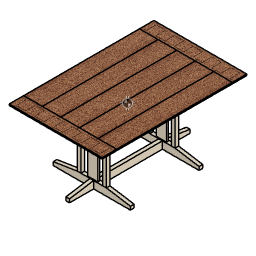
Trestle Table 2020 (Autodesk Fusion 360 design; units mm, degrees)
Autodesk Fusion 360 part; units mm, degrees
(part 1 of 2)
sketch "Sketch2" plane through (0, 0, 0) normal (1, 0, 0) x (0, 1, 0) in component "TopBoard"
  line L0 (0, 0) -> (1219.2, 0)
  line L1 (1219.2, 22.225) -> (0, 22.225)
  line L2 (609.6, 22.225) -> (609.6, 0) construction
  line L3 (0, 14.2875) -> (-25.4, 14.2875)
  line L4 (-25.4, 14.2875) -> (-25.4, 7.9375)
  line L5 (-25.4, 7.9375) -> (0, 7.9375)
  line L6 (0, 22.225) -> (0, 14.2875)
  line L7 (0, 7.9375) -> (0, 0)
  line L8 (1244.6, 14.2875) -> (1244.6, 7.9375)
  line L9 (1219.2, 22.225) -> (1219.2, 14.2875)
  line L10 (1244.6, 7.9375) -> (1219.2, 7.9375)
  line L11 (1219.2, 7.9375) -> (1219.2, 0)
  line L12 (1219.2, 14.2875) -> (1244.6, 14.2875)
  line L13 (1219.2, 0) -> (1219.2, 22.225) construction
  dimension "d18" = 1219.2
  dimension "d19" = 22.225
  dimension "d20" = 25.4
  dimension "d21" = 6.35
  constraint horizontal L0
  constraint horizontal L1
  constraint vertical L6
  constraint coincident L0.start L7.end
  constraint midpoint L1 L2.start
  constraint midpoint L0 L2.end
  constraint perpendicular L3 L6
  constraint perpendicular L3 L4
  constraint coincident L5.end L6
  constraint perpendicular L5 L6
  constraint collinear L6 L7
  constraint equal L6 L7
  constraint symmetric L0.start L2 L0.end
  constraint symmetric L1.end L2 L1.start
  constraint symmetric L2 L3.start L9.end
  constraint symmetric L2 L3.end L8.start
  constraint symmetric L2 L4.end L8.end
  constraint symmetric L2 L5.end L10.end
  constraint perpendicular L0 L13
  measures "d18" distance of L0.start L0.end
  measures "d19" distance of L0 L1
  measures "d20" distance of L3.start L3.end
  measures "d21" distance of L3.end L4.end
extrude "Extrude1" add sketch "Sketch2" along normal blind 195.58 makes body 1 in component "TopBoard"
ref_plane "WorkPlane1" through (97.79, 609.6, 11.1125) normal (0, -1, 0) x (0, 0, -1) in component "TopBoard"
sketch "Sketch3" plane through (0, -25.4, 0) normal (0, -1, 0) x (1, 0, 0) in component "TopBoard"
  line L0 (0, 14.2875) -> (0, 7.9375)
  line L1 (0, 7.9375) -> (195.58, 7.9375)
  line L2 (195.58, 7.9375) -> (195.58, 14.2875)
  line L3 (195.58, 14.2875) -> (0, 14.2875)
  line L4 (48.895, 14.2875) -> (146.685, 14.2875)
  line L5 (146.685, 14.2875) -> (146.685, 7.9375)
  line L6 (146.685, 7.9375) -> (48.895, 7.9375)
  line L7 (48.895, 7.9375) -> (48.895, 14.2875)
  dimension "d28" = 97.79
  constraint horizontal L4
  constraint vertical L5
  constraint horizontal L6
  constraint vertical L7
  constraint coincident L1 L5.end
  constraint coincident L3 L4.start
  constraint midpoint L3 L4
  measures "d28" distance of L4.start L4.end
extrude "Extrude2" add sketch "Sketch3" along normal blind 101.6 contours L1 L3 L4 L5 L6 L7 bodies 1 in component "TopBoard"
mirror "Mirror1" about plane through (97.79, 609.6, 11.1125) normal (0, -1, 0) of "Extrude2" in component "TopBoard"
sketch "Sketch4" plane through (0, 0, 0) normal (-1, 0, 0) x (0, -1, 0) in component "TopBoard"
  line L0 (0, 22.225) -> (-1219.2, 22.225)
  line L1 (-1219.2, 22.225) -> (-1219.2, 14.2875)
  line L2 (-1219.2, 14.2875) -> (-1244.6, 14.2875)
  line L3 (-1244.6, 14.2875) -> (-1244.6, 7.9375)
  line L4 (-1244.6, 7.9375) -> (-1219.2, 7.9375)
  line L5 (-1219.2, 7.9375) -> (-1219.2, 0)
  line L6 (-1219.2, 0) -> (0, 0)
  line L7 (0, 0) -> (0, 7.9375)
  line L8 (0, 7.9375) -> (25.4, 7.9375)
  line L9 (25.4, 7.9375) -> (25.4, 14.2875)
  line L10 (25.4, 14.2875) -> (0, 14.2875)
  line L11 (0, 14.2875) -> (0, 22.225)
  line L12 (-264.1209, 0) -> (-266.7, 7.9375)
  line L13 (-266.7, 7.9375) -> (-228.6, 7.9375)
  line L14 (-228.6, 7.9375) -> (-231.1791, 0)
  dimension "d61" = 38.1
  dimension "d62" = 108
  dimension "d63" = 108
  dimension "d64" = 7.9375
  dimension "d65" = 228.6
  constraint coincident L6 L12.start
  constraint parallel L6 L13
  constraint coincident L6 L14.end
  measures "d61" distance of L12.end L13.end
  measures "d62" angle of L6 L12
  measures "d63" angle of L6 L14
  measures "d64" distance of L6 L13
  measures "d65" distance of L7 L13.end
extrude "Extrude3" cut sketch "Sketch4" against normal up to surface (195.58 mm away) contours L6 L12 L13 L14 bodies 1 in component "TopBoard"
mirror "Mirror5" about plane through (97.79, 609.6, 11.1125) normal (0, -1, 0) of "Extrude3" in component "TopBoard"
pattern_linear "00000000-0000-0000-0000-000000000000" [suppressed]
sketch "Sketch2 (2)" plane through (0, 0, 0) normal (1, 0, 0) x (0, 1, 0) in component "TopBoard_Edge"
  line L0 (0, 0) -> (1219.2, 0)
  line L1 (1219.2, 22.225) -> (0, 22.225)
  line L2 (609.6, 22.225) -> (609.6, 0) construction
  line L3 (0, 14.2875) -> (-25.4, 14.2875)
  line L4 (-25.4, 14.2875) -> (-25.4, 7.9375)
  line L5 (-25.4, 7.9375) -> (0, 7.9375)
  line L6 (0, 22.225) -> (0, 14.2875)
  line L7 (0, 7.9375) -> (0, 0)
  line L8 (1244.6, 14.2875) -> (1244.6, 7.9375)
  line L9 (1219.2, 22.225) -> (1219.2, 14.2875)
  line L10 (1244.6, 7.9375) -> (1219.2, 7.9375)
  line L11 (1219.2, 7.9375) -> (1219.2, 0)
  line L12 (1219.2, 14.2875) -> (1244.6, 14.2875)
  line L13 (1219.2, 0) -> (1219.2, 22.225) construction
  dimension "d18_1" = 1219.2
  dimension "d19_1" = 22.225
  dimension "d20_1" = 25.4
  dimension "d21_1" = 6.35
  constraint horizontal L0
  constraint horizontal L1
  constraint vertical L6
  constraint coincident L0.start L7.end
  constraint midpoint L1 L2.start
  constraint midpoint L0 L2.end
  constraint perpendicular L3 L6
  constraint perpendicular L3 L4
  constraint coincident L5.end L6
  constraint perpendicular L5 L6
  constraint collinear L6 L7
  constraint equal L6 L7
  constraint symmetric L0.start L2 L0.end
  constraint symmetric L1.end L2 L1.start
  constraint symmetric L2 L3.start L9.end
  constraint symmetric L2 L3.end L8.start
  constraint symmetric L2 L4.end L8.end
  constraint symmetric L2 L5.end L10.end
  constraint perpendicular L0 L13
  measures "d18_1" distance of L0.start L0.end
  measures "d19_1" distance of L0 L1
  measures "d20_1" distance of L3.start L3.end
  measures "d21_1" distance of L3.end L4.end
extrude "Extrude1'" add sketch "Sketch2 (2)" along normal blind 195.58 separate body makes body 2 in component "TopBoard_Edge"
ref_plane "WorkPlane1" through (97.79, 609.6, 11.1125) normal (0, -1, 0) x (0, 0, -1) in component "TopBoard_Edge"
sketch "Sketch3 (2)" plane through (0, -25.4, 0) normal (0, -1, 0) x (1, 0, 0) in component "TopBoard_Edge"
  line L0 (0, 14.2875) -> (0, 7.9375)
  line L1 (0, 7.9375) -> (195.58, 7.9375)
  line L2 (195.58, 7.9375) -> (195.58, 14.2875)
  line L3 (195.58, 14.2875) -> (0, 14.2875)
  line L4 (48.895, 14.2875) -> (146.685, 14.2875)
  line L5 (146.685, 14.2875) -> (146.685, 7.9375)
  line L6 (146.685, 7.9375) -> (48.895, 7.9375)
  line L7 (48.895, 7.9375) -> (48.895, 14.2875)
  dimension "d28_1" = 97.79
  constraint horizontal L4
  constraint vertical L5
  constraint horizontal L6
  constraint vertical L7
  constraint coincident L1 L5.end
  constraint coincident L3 L4.start
  constraint midpoint L3 L4
  measures "d28_1" distance of L4.start L4.end
extrude "Extrude2'" add sketch "Sketch3 (2)" along normal blind 101.6 contours L1 L3 L4 L5 L6 L7 bodies 2 in component "TopBoard_Edge"
mirror "Mirror1'" about plane through (97.79, 609.6, 11.1125) normal (0, -1, 0) of "Extrude2'" in component "TopBoard_Edge"
sketch "Sketch4 (2)" plane through (0, 0, 0) normal (-1, 0, 0) x (0, -1, 0) in component "TopBoard_Edge"
  line L0 (0, 22.225) -> (-1219.2, 22.225)
  line L1 (-1219.2, 22.225) -> (-1219.2, 14.2875)
  line L2 (-1219.2, 14.2875) -> (-1244.6, 14.2875)
  line L3 (-1244.6, 14.2875) -> (-1244.6, 7.9375)
  line L4 (-1244.6, 7.9375) -> (-1219.2, 7.9375)
  line L5 (-1219.2, 7.9375) -> (-1219.2, 0)
  line L6 (-1219.2, 0) -> (0, 0)
  line L7 (0, 0) -> (0, 7.9375)
  line L8 (0, 7.9375) -> (25.4, 7.9375)
  line L9 (25.4, 7.9375) -> (25.4, 14.2875)
  line L10 (25.4, 14.2875) -> (0, 14.2875)
  line L11 (0, 14.2875) -> (0, 22.225)
  line L12 (-264.1209, 0) -> (-266.7, 7.9375)
  line L13 (-266.7, 7.9375) -> (-228.6, 7.9375)
  line L14 (-228.6, 7.9375) -> (-231.1791, 0)
  dimension "d61_1" = 38.1
  dimension "d62_1" = 108
  dimension "d63_1" = 108
  dimension "d64_1" = 7.9375
  dimension "d65_1" = 228.6
  constraint coincident L6 L12.start
  constraint parallel L6 L13
  constraint coincident L6 L14.end
  measures "d61_1" distance of L12.end L13.end
  measures "d62_1" angle of L6 L12
  measures "d63_1" angle of L6 L14
  measures "d64_1" distance of L6 L13
  measures "d65_1" distance of L7 L13.end
extrude "Extrude3'" cut sketch "Sketch4 (2)" against normal up to surface (195.58 mm away) contours L6 L12 L13 L14 bodies 2 in component "TopBoard_Edge"
mirror "Mirror5'" about plane through (97.79, 609.6, 11.1125) normal (0, -1, 0) of "Extrude3'" in component "TopBoard_Edge"
chamfer "Chamfer1" distance 50.1154 angle 9 3 edges at (0, 609.6, 0) (0, 115.5895, 0) (0, 1103.6105, 0) measured on face at (65.1933, 494.4403, 0) measured on face at (65.1933, 154.1194, 0) measured on face at (65.1933, 1065.0806, 0) on bodies 2 in component "TopBoard_Edge"
sketch "Sketch1" plane through (0, 0, 0) normal (1, 0, 0) x (0, 1, 0) in component "BreadBoard"
  line L0 (50.1154, 0) -> (152.4, 0)
  line L1 (152.4, 22.225) -> (0, 22.225)
  line L2 (0, 22.225) -> (0, 7.9375)
  line L3 (152.4, 14.2875) -> (127, 14.2875)
  line L4 (127, 14.2875) -> (127, 7.9375)
  line L5 (127, 7.9375) -> (152.4, 7.9375)
  line L6 (152.4, 0) -> (152.4, 7.9375)
  line L7 (152.4, 14.2875) -> (152.4, 22.225)
  line L8 (0, 7.9375) -> (50.1154, 0)
  dimension "d99" = 22.225
  dimension "d100" = 7.9375
  dimension "d103" = 152.4
  dimension "d104" = 6.35
  dimension "d105" = 25.4
  dimension "d596" = 99
  constraint horizontal L0
  constraint vertical L6
  constraint horizontal L1
  constraint vertical L2
  constraint coincident L3.start L6
  constraint perpendicular L3 L6
  constraint perpendicular L3 L4
  constraint perpendicular L5 L6
  constraint collinear L6 L7
  constraint equal L6 L7
  constraint coincident origin L2
  constraint coincident origin L0
  measures "d99" distance of origin L1.end
  measures "d100" distance of L0 L2.end
  measures "d103" distance of L1.start L1.end
  measures "d104" distance of L3.end L4.end
  measures "d105" distance of L3.start L3.end
  measures "d596" angle of L2 L8
extrude "Extrude1''" add sketch "Sketch1" along normal blind 977.9 separate body makes body 3 in component "BreadBoard"
sketch "Sketch2 (3)" plane through (0, 127, 0) normal (0, 1, 0) x (-1, 0, 0) in component "BreadBoard"
  line L0 (0, 7.9375) -> (0, 14.2875)
  line L1 (0, 14.2875) -> (-977.9, 14.2875)
  line L2 (-977.9, 14.2875) -> (-977.9, 7.9375)
  line L3 (-977.9, 7.9375) -> (0, 7.9375)
  line L4 (-146.685, 14.2875) -> (-48.895, 14.2875)
  line L5 (-48.895, 14.2875) -> (-48.895, 7.9375)
  line L6 (-48.895, 7.9375) -> (-146.685, 7.9375)
  line L7 (-146.685, 7.9375) -> (-146.685, 14.2875)
  line L8 (-342.265, 7.9375) -> (-342.265, 14.2875)
  line L9 (-244.475, 14.2875) -> (-244.475, 7.9375)
  line L10 (-244.475, 7.9375) -> (-342.265, 7.9375)
  line L11 (-342.265, 14.2875) -> (-244.475, 14.2875)
  line L12 (-537.845, 7.9375) -> (-537.845, 14.2875)
  line L13 (-440.055, 14.2875) -> (-440.055, 7.9375)
  line L14 (-440.055, 7.9375) -> (-537.845, 7.9375)
  line L15 (-537.845, 14.2875) -> (-440.055, 14.2875)
  line L16 (-733.425, 7.9375) -> (-733.425, 14.2875)
  line L17 (-635.635, 14.2875) -> (-635.635, 7.9375)
  line L18 (-635.635, 7.9375) -> (-733.425, 7.9375)
  line L19 (-733.425, 14.2875) -> (-635.635, 14.2875)
  line L20 (-929.005, 7.9375) -> (-929.005, 14.2875)
  line L21 (-831.215, 14.2875) -> (-831.215, 7.9375)
  line L22 (-831.215, 7.9375) -> (-929.005, 7.9375)
  line L23 (-929.005, 14.2875) -> (-831.215, 14.2875)
  dimension "d108" = 97.79
  dimension "d109" = 48.895
  dimension "d113" = 195.58
  dimension "d114" = 0
  constraint horizontal L4
  constraint vertical L5
  constraint horizontal L6
  constraint vertical L7
  constraint coincident L3 L5.end
  constraint coincident L1 L4.start
  measures "d108" distance of L4.start L4.end
  measures "d109" distance of L0 L5
extrude "Extrude2''" cut sketch "Sketch2 (3)" against normal blind 101.6 contours L1 L3 L4 L5 L6 L7 | L1 L3 L8 L9 L10 L11 | L1 L3 L12 L13 L14 L15 | L1 L3 L16 L17 L18 L19 | L1 L3 L20 L21 L22 L23 bodies 3 in component "BreadBoard"
sketch "Sketch3 (3)" plane through (0, 152.4, 0) normal (0, 1, 0) x (-1, 0, 0) in component "BreadBoard"
  line L0 (0, 0) -> (0, 7.9375)
  line L1 (0, 7.9375) -> (-977.9, 7.9375)
  line L2 (-977.9, 7.9375) -> (-977.9, 0)
  line L3 (-977.9, 0) -> (0, 0)
  line L4 (0, 7.9375) -> (-50.1154, 0)
  line L5 (0, 14.2875) -> (0, 7.9375)
  dimension "d118" = 7.9375
  dimension "d597" = 99
  constraint coincident L3 L4.end
  constraint coincident L0 L1.start
  measures "d118" distance of L0.start L0.end
  measures "d597" angle of L4 L5
ref_plane "WorkPlane1" through (488.95, 76.2, 11.1125) normal (-1, 0, 0) x (0, -1, 0) in component "BreadBoard"
extrude "Extrude3''" cut sketch "Sketch3 (3)" against normal up to surface (152.4 mm away) contours L0 L3 L4 bodies 3 in component "BreadBoard"
mirror "Mirror1''" about plane through (488.95, 76.2, 11.1125) normal (-1, 0, 0) of "Extrude3''" in component "BreadBoard"
sketch "Sketch1 (2)" plane through (0, 0, 0) normal (1, 0, 0) x (0, 1, 0) in component "TrestleTop"
  line L0 (0, 0) -> (38.1, 0)
  line L1 (38.1, 0) -> (38.1, 76.2)
  line L2 (0, 76.2) -> (0, 0)
  line L3 (38.1, 76.2) -> (35.5209, 76.2)
  line L4 (2.5791, 76.2) -> (0, 76.2)
  line L5 (2.5791, 76.2) -> (0, 84.1375)
  line L6 (0, 84.1375) -> (38.1, 84.1375)
  line L7 (38.1, 84.1375) -> (35.5209, 76.2)
  dimension "d146" = 76.2
  dimension "d147" = 38.1
  dimension "d148" = 7.9375
  dimension "d149" = 72
  constraint horizontal L0
  constraint vertical L1
  constraint horizontal L3
  constraint vertical L2
  constraint coincident L0.start L2.end
  constraint coincident L4.start L3
  constraint collinear L3 L4
  constraint equal L3 L4
  constraint parallel L4 L6
  constraint coincident L1 L6.end
  constraint coincident L2 L5.end
  measures "d146" distance of L0.start L2.start
  measures "d147" distance of L0.start L0.end
  measures "d148" distance of L4 L6
  measures "d149" angle of L5 L6
extrude "Extrude1'''" add sketch "Sketch1 (2)" along normal blind 812.8 separate body makes body 4 in component "TrestleTop"
sketch "Sketch2 (4)" plane through (0, 0, 0) normal (0, -1, 0) x (1, 0, 0) in component "TrestleTop"
  line L0 (0, 76.2) -> (0, 0)
  line L1 (0, 0) -> (812.8, 0)
  line L2 (812.8, 0) -> (812.8, 76.2)
  line L3 (812.8, 76.2) -> (0, 76.2)
  line L4 (0, 40.2296) -> (254, 0)
  line L5 (406.4, 76.2) -> (406.4, 0) construction
  line L6 (812.8, 40.2296) -> (558.8, 0)
  dimension "d158" = 9
  dimension "d159" = 304.8
  dimension "d161" = 35.9704
  constraint coincident L0 L4.start
  constraint coincident L1 L4.end
  constraint midpoint L3 L5.start
  constraint midpoint L1 L5.end
  constraint symmetric L4.start L5 L6.start
  constraint symmetric L4.end L5 L6.end
  measures "d158" angle of L1 L4
  measures "d159" distance of L4.end L6.end
  measures "d161" distance of L0.start L4.start
extrude "Extrude2'''" cut sketch "Sketch2 (4)" against normal up to surface (38.1 mm away) contours L0 L1 L4 | L1 L2 L6 bodies 4 in component "TrestleTop"
sketch "Sketch3 (4)" plane through (0, 0, 0) normal (0, 0, -1) x (1, 0, 0) in component "TrestleTop"
  line L0 (254, 0) -> (254, -38.1)
  line L1 (254, -38.1) -> (558.8, -38.1)
  line L2 (558.8, -38.1) -> (558.8, 0)
  line L3 (558.8, 0) -> (254, 0)
  line L4 (260.35, -12.7) -> (285.75, -12.7)
  line L5 (285.75, -12.7) -> (285.75, -25.4)
  line L6 (285.75, -25.4) -> (260.35, -25.4)
  line L7 (260.35, -25.4) -> (260.35, -12.7)
  line L8 (285.7253, 0) -> (285.7747, -38.1) construction
  line L9 (406.4, 0) -> (406.4, -38.1) construction
  line L10 (552.45, -12.7) -> (527.05, -12.7)
  line L11 (552.45, -25.4) -> (552.45, -12.7)
  line L12 (527.05, -25.4) -> (552.45, -25.4)
  line L13 (527.05, -12.7) -> (527.05, -25.4)
  line L14 (355.9175, -12.7) -> (456.8825, -12.7)
  line L15 (456.8825, -12.7) -> (456.8825, -25.4)
  line L16 (456.8825, -25.4) -> (355.9175, -25.4)
  line L17 (355.9175, -25.4) -> (355.9175, -12.7)
  line L18 (456.8825, -12.7) -> (355.9175, -25.4) construction
  dimension "d162" = 6.35
  dimension "d163" = 25.4
  dimension "d164" = 12.7
  dimension "d592" = 12.7
  dimension "d593" = 100.965
  constraint vertical L5
  constraint vertical L7
  constraint coincident L3 L8.start
  constraint coincident L1 L8.end
  constraint midpoint L5 L8
  constraint midpoint L3 L9.start
  constraint midpoint L1 L9.end
  constraint symmetric L4.start L9 L10.start
  constraint symmetric L4.end L9 L10.end
  constraint symmetric L5.end L9 L12.start
  constraint symmetric L6.end L9 L11.start
  constraint horizontal L14
  constraint vertical L15
  constraint horizontal L16
  constraint vertical L17
  constraint midpoint L9 L18
  constraint horizontal L4
  constraint horizontal L6
  measures "d162" distance of L0 L7
  measures "d163" distance of L4.start L4.end
  measures "d164" distance of L4.start L6.end
  measures "d592" distance of L14.end L15.end
  measures "d593" distance of L14.start L14.end
extrude "Extrude3'''" cut sketch "Sketch3 (4)" against normal blind 38.1 contours L4 L5 L6 L7 | L10 L11 L12 L13 bodies 4 in component "TrestleTop"
sketch "Sketch1 (3)" plane through (0, 0, 0) normal (0, 0, 1) x (1, 0, 0) in component "TrestlePost"
  line L0 (0, 0) -> (38.1, 0)
  line L1 (38.1, 0) -> (38.1, 38.1)
  line L2 (38.1, 38.1) -> (0, 38.1)
  line L3 (0, 38.1) -> (0, 0)
  dimension "d199" = 38.1
  constraint horizontal L0
  constraint vertical L1
  constraint horizontal L2
  constraint vertical L3
  constraint coincident L0.start L3.end
  constraint equal L1 L2
  measures "d199" distance of L0.end L1.end
extrude "Extrude1''''" add sketch "Sketch1 (3)" along normal blind 536.575 separate body makes body 5 in component "TrestlePost"
ref_plane "WorkPlane1" through (19.05, 19.05, 268.2875) normal (0, 0, 1) x (1, 0, 0) in component "TrestlePost"
sketch "Sketch2 (5)" plane through (0, 0, 536.575) normal (0, 0, 1) x (-1, 0, 0) in component "TrestlePost"
  line L0 (0, -38.1) -> (0, 0)
  line L1 (0, 0) -> (-38.1, 0)
  line L2 (-38.1, 0) -> (-38.1, -38.1)
  line L3 (-38.1, -38.1) -> (0, -38.1)
  line L4 (-6.35, -25.4) -> (-31.75, -25.4)
  line L5 (-31.75, -25.4) -> (-31.75, -12.7)
  line L6 (-31.75, -12.7) -> (-6.35, -12.7)
  line L7 (-6.35, -12.7) -> (-6.35, -25.4)
  line L8 (0, -38.1) -> (-38.1, 0) construction
  line L9 (-31.75, -25.4) -> (-6.35, -12.7) construction
  dimension "d202" = 12.7
  dimension "d203" = 6.35
  constraint horizontal L4
  constraint vertical L5
  constraint horizontal L6
  constraint vertical L7
  constraint coincident L0.start L3.end
  constraint coincident L1.end L2.start
  constraint midpoint L8 L9
  measures "d202" distance of L4.end L5.end
  measures "d203" distance of L2 L5
extrude "Extrude2''''" add sketch "Sketch2 (5)" along normal blind 38.1 contours L4 L5 L6 L7 bodies 5 in component "TrestlePost"
mirror "Mirror1'''" about plane through (19.05, 19.05, 268.2875) normal (0, 0, 1) of "Extrude2''''" in component "TrestlePost"
sketch "Sketch1 (4)" plane through (0, 0, 0) normal (1, 0, 0) x (0, 1, 0) in component "TrestleBase"
  line L0 (0, 0) -> (38.1, 0)
  line L1 (38.1, 0) -> (38.1, 76.2)
  line L2 (0, 76.2) -> (0, 0)
  line L3 (38.1, 76.2) -> (0, 76.2)
  dimension "d146_1" = 76.2
  dimension "d147_1" = 38.1
  dimension "d572" = 0
  dimension "d573" = 0
  dimension "d574" = 0
  dimension "d575" = 0
  dimension "d584" = 0
  dimension "d585" = 0
  dimension "d586" = 0
  dimension "d587" = 0
  constraint horizontal L0
  constraint vertical L1
  constraint vertical L2
  constraint coincident L0.start L2.end
  constraint horizontal L3
  measures "d146_1" distance of L0.start L2.start
  measures "d147_1" distance of L0.start L0.end
extrude "Extrude1'''''" add sketch "Sketch1 (4)" along normal blind 812.8 separate body makes body 6 in component "TrestleBase"
sketch "Sketch2 (6)" plane through (0, 0, 0) normal (0, -1, 0) x (1, 0, 0) in component "TrestleBase"
  line L0 (0, 76.2) -> (0, 0)
  line L1 (0, 0) -> (812.8, 0)
  line L2 (812.8, 0) -> (812.8, 76.2)
  line L3 (0, 40.2296) -> (254, 0)
  line L4 (406.4, 76.2) -> (406.4, 0) construction
  line L5 (812.8, 40.2296) -> (558.8, 0)
  line L6 (812.8, 76.2) -> (0, 76.2)
  line L7 (425.45, 76.2) -> (425.45, 38.1)
  line L8 (425.45, 38.1) -> (387.35, 38.1)
  line L9 (387.35, 38.1) -> (387.35, 76.2)
  dimension "d158_1" = 9
  dimension "d159_1" = 304.8
  dimension "d161_1" = 35.9704
  dimension "d628" = 38.1
  constraint coincident L0 L3.start
  constraint coincident L1 L3.end
  constraint midpoint L1 L4.end
  constraint symmetric L3.start L4 L5.start
  constraint symmetric L3.end L4 L5.end
  constraint coincident L1 L5.end
  constraint coincident L6 L7.start
  constraint perpendicular L6 L7
  constraint perpendicular L7 L8
  constraint coincident L6 L9.end
  constraint perpendicular L6 L9
  constraint midpoint L4 L8
  constraint coincident L4.start L6
  measures "d158_1" angle of L1 L3
  measures "d159_1" distance of L3.end L5.end
  measures "d161_1" distance of L0.start L3.start
  measures "d628" distance of L7.start L9.end
extrude "Extrude2'''''" cut sketch "Sketch2 (6)" against normal up to surface (38.1 mm away) contours L0 L1 L3 | L6 L7 L8 L9 | L1 L2 L5 bodies 6 in component "TrestleBase"
sketch "Sketch3 (5)" plane through (0, 0, 0) normal (0, 0, -1) x (1, 0, 0) in component "TrestleBase"
  line L0 (254, 0) -> (254, -38.1)
  line L1 (254, -38.1) -> (558.8, -38.1)
  line L2 (558.8, -38.1) -> (558.8, 0)
  line L3 (558.8, 0) -> (254, 0)
  line L4 (260.35, -12.7) -> (285.75, -12.7)
  line L5 (285.75, -12.7) -> (285.75, -25.4)
  line L6 (285.75, -25.4) -> (260.35, -25.4)
  line L7 (260.35, -25.4) -> (260.35, -12.7)
  line L8 (285.7946, 0) -> (285.7054, -38.1) construction
  line L9 (406.4, 0) -> (406.4, -38.1) construction
  line L10 (552.45, -12.7) -> (527.05, -12.7)
  line L11 (552.45, -25.4) -> (552.45, -12.7)
  line L12 (527.05, -25.4) -> (552.45, -25.4)
  line L13 (527.05, -12.7) -> (527.05, -25.4)
  line L14 (355.9175, -12.7) -> (456.8825, -12.7)
  line L15 (456.8825, -12.7) -> (456.8825, -25.4)
  line L16 (456.8825, -25.4) -> (355.9175, -25.4)
  line L17 (355.9175, -25.4) -> (355.9175, -12.7)
  line L18 (456.8825, -12.7) -> (355.9175, -25.4) construction
  dimension "d162_1" = 6.35
  dimension "d163_1" = 25.4
  dimension "d164_1" = 12.7
  dimension "d559" = 100.965
  dimension "d560" = 12.7
  constraint vertical L5
  constraint vertical L7
  constraint coincident L3 L8.start
  constraint coincident L1 L8.end
  constraint midpoint L5 L8
  constraint midpoint L3 L9.start
  constraint midpoint L1 L9.end
  constraint symmetric L4.start L9 L10.start
  constraint symmetric L4.end L9 L10.end
  constraint symmetric L5.end L9 L12.start
  constraint symmetric L6.end L9 L11.start
  constraint horizontal L14
  constraint vertical L15
  constraint horizontal L16
  constraint vertical L17
  constraint horizontal L4
  constraint horizontal L6
  constraint midpoint L9 L18
  measures "d162_1" distance of L0 L7
  measures "d163_1" distance of L4.start L4.end
  measures "d164_1" distance of L4.start L6.end
  measures "d559" distance of L14.start L14.end
  measures "d560" distance of L14.end L15.end
extrude "Extrude3''''" cut sketch "Sketch3 (5)" against normal blind 38.1 contours L4 L5 L6 L7 | L10 L11 L12 L13 bodies 6 in component "TrestleBase"
sketch "Sketch3 (6)" plane through (0, 0, 0) normal (0, -1, 0) x (1, 0, 0) in component "TrestlePost"
  line L0 (0, 0) -> (38.1, 0)
  line L1 (38.1, 0) -> (38.1, 536.575)
  line L2 (38.1, 536.575) -> (0, 536.575)
  line L3 (0, 536.575) -> (0, 0)
  line L4 (12.7, 479.425) -> (25.4, 479.425)
  line L5 (25.4, 479.425) -> (25.4, 377.825)
  line L6 (25.4, 377.825) -> (12.7, 377.825)
  line L7 (12.7, 377.825) -> (12.7, 479.425)
  line L8 (0, 479.425) -> (38.1, 479.425) construction
  dimension "d337" = 12.7
  dimension "d338" = 101.6
  dimension "d339" = 377.825
  constraint horizontal L4
  constraint vertical L5
  constraint horizontal L6
  constraint vertical L7
  constraint coincident L3 L8.start
  constraint coincident L1 L8.end
  constraint perpendicular L1 L8
  constraint midpoint L4 L8
  measures "d337" distance of L4.start L4.end
  measures "d338" distance of L4.start L6.end
  measures "d339" distance of L0 L6
extrude "Extrude3'''''" cut sketch "Sketch3 (6)" against normal up to surface (38.1 mm away) contours L4 L5 L6 L7 bodies 5 in component "TrestlePost"
sketch "Sketch1 (5)" plane through (0, 0, 0) normal (0, 1, 0) x (1, 0, 0) in component "Stretcher"
  line L0 (0, 0) -> (19.304, 0)
  line L1 (19.304, 0) -> (19.304, -114.3)
  line L2 (19.304, -114.3) -> (0, -114.3)
  line L3 (0, -114.3) -> (0, 0)
  dimension "d366" = 19.304
  dimension "d367" = 114.3
  constraint horizontal L0
  constraint vertical L1
  constraint horizontal L2
  constraint vertical L3
  constraint coincident L0.start L3.end
  measures "d366" distance of L0.start L0.end
  measures "d367" distance of L0.start L2.end
extrude "Extrude1''''''" add sketch "Sketch1 (5)" along normal blind 685.8 separate body makes body 7 in component "Stretcher"
ref_plane "WorkPlane1" through (9.652, 342.9, 57.15) normal (0, 1, 0) x (0, 0, 1) in component "Stretcher"
sketch "Sketch2 (7)" plane through (0, 0, 0) normal (0, -1, 0) x (1, 0, 0) in component "Stretcher"
  line L0 (19.304, 114.3) -> (0, 114.3)
  line L1 (0, 114.3) -> (0, 0)
  line L2 (0, 0) -> (19.304, 0)
  line L3 (19.304, 0) -> (19.304, 114.3)
  line L4 (3.302, 107.95) -> (16.002, 107.95)
  line L5 (16.002, 107.95) -> (16.002, 6.35)
  line L6 (16.002, 6.35) -> (3.302, 6.35)
  line L7 (3.302, 6.35) -> (3.302, 107.95)
  line L8 (0, 114.3) -> (19.304, 0) construction
  line L9 (3.302, 6.35) -> (16.002, 107.95) construction
  dimension "d370" = 6.35
  dimension "d372" = 12.7
  constraint horizontal L4
  constraint vertical L5
  constraint horizontal L6
  constraint vertical L7
  constraint coincident L0.end L1.start
  constraint coincident L2.end L3.start
  constraint midpoint L8 L9
  measures "d370" distance of L0 L4
  measures "d372" distance of L4.start L4.end
extrude "Extrude2''''''" add sketch "Sketch2 (7)" along normal blind 38.1 contours L4 L5 L6 L7 bodies 7 in component "Stretcher"
ref_plane "WorkPlane2" through (9.652, -19.05, 57.15) normal (1, 0, 0) x (0, 0, 1) in component "Stretcher"
sketch "Sketch3 (7)" plane through (9.652, -50.8, 38.1) normal (1, 0, 0) x (0, 1, 0) in component "Stretcher"
  line L0 (50.8, 69.85) -> (12.7, 69.85)
  line L1 (50.8, -31.75) -> (12.7, -31.75)
  line L2 (12.7, 69.85) -> (12.7, -31.75)
  line L3 (12.7, -31.75) -> (0, -31.75)
  line L4 (0, -31.75) -> (-7.9961, 69.85)
  line L5 (-7.9961, 69.85) -> (12.7, 69.85)
  line L6 (50.8, 76.2) -> (50.8, -38.1)
  dimension "d400" = 38.1
  dimension "d401" = 4.5
  dimension "d404" = 12.7
  constraint coincident L0 L2.start
  constraint coincident L1 L2.end
  constraint perpendicular L1 L2
  constraint coincident L0 L4.end
  constraint coincident L1 L3.end
  measures "d400" distance of L2 L6
  measures "d401" angle of L2 L4
  measures "d404" distance of L1.end L3.end
mirror "Mirror2" about plane through (9.652, 342.9, 57.15) normal (0, 1, 0) of "Extrude2''''''" in component "Stretcher"
sketch "Sketch1 (6)" plane through (0, 0, 0) normal (0, 1, 0) x (1, 0, 0) in component "Panel"
  line L0 (140.97, 76.2) -> (445.77, 76.2)
  line L1 (140.97, 612.775) -> (445.77, 612.775)
  line L2 (252.9511, 76.2) -> (360.2661, 76.2)
  line L3 (360.2661, 76.2) -> (360.2661, 612.775)
  line L4 (360.2661, 612.775) -> (252.9511, 612.775)
  line L5 (252.9511, 612.775) -> (252.9511, 76.2)
  dimension "d530" = 107.315
  dimension "d568" = 0
  dimension "d569" = 0
  dimension "d570" = 0
  dimension "d571" = 0
  dimension "d580" = 0
  dimension "d581" = 0
  dimension "d582" = 0
  dimension "d583" = 0
  constraint horizontal L2
  constraint vertical L3
  constraint horizontal L4
  constraint vertical L5
  constraint coincident L1 L3.end
  constraint coincident L0 L2.start
  measures "d530" distance of L3.end L4.end
extrude "Extrude1'''''''" add sketch "Sketch1 (6)" along normal blind 19.304 separate body makes body 8 in component "Panel"
ref_plane "WorkPlane1" through (306.6086, 9.652, -344.4875) normal (0, 0, 1) x (1, 0, 0) in component "Panel"
sketch "Sketch2 (8)" plane through (0, 0, -76.2) normal (0, 0, 1) x (-1, 0, 0) in component "Panel"
  line L0 (-252.9511, 0) -> (-360.2661, 0)
  line L1 (-360.2661, 0) -> (-360.2661, -19.304)
  line L2 (-360.2661, -19.304) -> (-252.9511, -19.304)
  line L3 (-252.9511, -19.304) -> (-252.9511, 0)
  line L4 (-256.1261, -16.002) -> (-357.0911, -16.002)
  line L5 (-357.0911, -16.002) -> (-357.0911, -3.302)
  line L6 (-357.0911, -3.302) -> (-256.1261, -3.302)
  line L7 (-256.1261, -3.302) -> (-256.1261, -16.002)
  line L8 (-256.1261, -3.302) -> (-357.0911, -16.002) construction
  line L9 (-306.6086, -19.304) -> (-306.6086, 0) construction
  dimension "d561" = 12.7
  dimension "d562" = 3.175
  constraint horizontal L4
  constraint vertical L5
  constraint horizontal L6
  constraint vertical L7
  constraint midpoint L2 L9.start
  constraint midpoint L0 L9.end
  constraint midpoint L8 L9
  measures "d561" distance of L4.end L5.end
  measures "d562" distance of L3 L7
extrude "Extrude2'''''''" add sketch "Sketch2 (8)" along normal blind 6.35 contours L4 L5 L6 L7 bodies 8 in component "Panel"
mirror "Mirror1''''" about plane through (306.6086, 9.652, -344.4875) normal (0, 0, 1) of "Extrude2'''''''" in component "Panel"
sketch "Sketch2 (9)" plane through (0, 0, 0) normal (0, 1, 0) x (1, 0, 0)
  line L0 (-113.03, 688.975) -> (293.37, 73.1846)
  line L1 (312.42, 688.975) -> (699.77, 688.975)
  line L2 (-113.03, 688.975) -> (274.32, 688.975)
extrude "Extrude4" cut sketch "Sketch3 (4)" against normal blind 6.35 contours L14 L15 L16 L17 bodies 4 in component "TrestleTop"
extrude "Extrude4'" cut sketch "Sketch3 (5)" against normal blind 6.35 contours L14 L15 L16 L17 bodies 6 in component "TrestleBase"
sketch "Sketch1 (7)" plane through (0, 0, 0) normal (1, 0, 0) x (0, 1, 0) in component "FloorStretcher"
  line L0 (0, 0) -> (1270, 0)
  line L1 (1270, 0) -> (1270, 35.9704)
  line L2 (1270, 35.9704) -> (1016, 76.2)
  line L3 (1016, 76.2) -> (1016, 38.1)
  line L4 (1016, 38.1) -> (977.9, 38.1)
  line L5 (977.9, 38.1) -> (977.9, 76.2)
  line L6 (977.9, 76.2) -> (292.1, 76.2)
  line L7 (292.1, 76.2) -> (292.1, 38.1)
  line L8 (292.1, 38.1) -> (254, 38.1)
  line L9 (254, 38.1) -> (254, 76.2)
  line L10 (254, 76.2) -> (0, 35.9704)
  line L11 (0, 35.9704) -> (0, 0)
  line L12 (1270, 35.9704) -> (0, 35.9704) construction
  line L13 (635, 76.2) -> (635, 0) construction
  dimension "d620" = 38.1
  dimension "d621" = 1270
  dimension "d622" = 38.1
  dimension "d623" = 9
  dimension "d624" = 76.2
  dimension "d625" = 762
  constraint coincident L0.start L11.end
  constraint horizontal L0
  constraint perpendicular L0 L1
  constraint perpendicular L3 L4
  constraint perpendicular L4 L5
  constraint perpendicular L3 L6
  constraint perpendicular L6 L7
  constraint perpendicular L7 L8
  constraint perpendicular L8 L9
  constraint horizontal L12
  constraint vertical L11
  constraint collinear L4 L8
  constraint equal L4 L8
  constraint midpoint L6 L13.start
  constraint midpoint L0 L13.end
  constraint vertical L13
  constraint coincident L2.end L6
  constraint coincident L6 L9.end
  measures "d620" distance of L0 L8
  measures "d621" distance of L0.start L0.end
  measures "d622" distance of L3.end L4.end
  measures "d623" angle of L10 L12
  measures "d624" distance of L0 L6
  measures "d625" distance of L2.end L9.end
extrude "Extrude1''''''''" add sketch "Sketch1 (7)" along normal blind 38.1 separate body makes body 9 in component "FloorStretcher"
sketch "Sketch3 (8)" plane through (0, 19.304, 0) normal (0, 1, 0) x (-1, 0, 0) in component "Panel"
  line L0 (-252.9511, -612.775) -> (-252.9511, -76.2)
  line L1 (-252.9511, -76.2) -> (-360.2661, -76.2)
  line L2 (-360.2661, -76.2) -> (-360.2661, -612.775)
  line L3 (-360.2661, -612.775) -> (-252.9511, -612.775)
  line L4 (-306.6086, -88.9) -> (-347.5661, -129.8575)
  line L5 (-347.5661, -129.8575) -> (-306.6086, -170.815)
  line L6 (-306.6086, -170.815) -> (-265.6511, -129.8575)
  line L7 (-265.6511, -129.8575) -> (-306.6086, -88.9)
  line L8 (-281.2086, -88.9) -> (-265.6511, -88.9)
  line L9 (-265.6511, -88.9) -> (-265.6511, -104.4575)
  line L10 (-265.6511, -104.4575) -> (-281.2086, -88.9)
  line L11 (-306.6086, -76.2) -> (-306.6086, -612.775) construction
  line L12 (-265.6511, -155.2575) -> (-293.9086, -183.515)
  line L13 (-293.9086, -183.515) -> (-265.6511, -211.7725)
  line L14 (-265.6511, -211.7725) -> (-265.6511, -155.2575)
  line L15 (-360.2661, -344.4875) -> (-252.9511, -344.4875) construction
  line L16 (-306.6086, -278.13) -> (-265.6511, -237.1725)
  line L17 (-347.5661, -237.1725) -> (-306.6086, -278.13)
  line L18 (-306.6086, -196.215) -> (-347.5661, -237.1725)
  line L19 (-265.6511, -237.1725) -> (-306.6086, -196.215)
  line L20 (-306.6086, -385.445) -> (-265.6511, -344.4875)
  line L21 (-347.5661, -344.4875) -> (-306.6086, -385.445)
  line L22 (-306.6086, -303.53) -> (-347.5661, -344.4875)
  line L23 (-265.6511, -344.4875) -> (-306.6086, -303.53)
  line L24 (-306.6086, -492.76) -> (-265.6511, -451.8025)
  line L25 (-347.5661, -451.8025) -> (-306.6086, -492.76)
  line L26 (-306.6086, -410.845) -> (-347.5661, -451.8025)
  line L27 (-265.6511, -451.8025) -> (-306.6086, -410.845)
  line L28 (-265.6511, -319.0875) -> (-265.6511, -262.5725)
  line L29 (-265.6511, -262.5725) -> (-293.9086, -290.83)
  line L30 (-293.9086, -290.83) -> (-265.6511, -319.0875)
  line L31 (-265.6511, -426.4025) -> (-265.6511, -369.8875)
  line L32 (-265.6511, -369.8875) -> (-293.9086, -398.145)
  line L33 (-293.9086, -398.145) -> (-265.6511, -426.4025)
  line L34 (-265.6511, -533.7175) -> (-265.6511, -477.2025)
  line L35 (-265.6511, -477.2025) -> (-293.9086, -505.46)
  line L36 (-293.9086, -505.46) -> (-265.6511, -533.7175)
  line L37 (-306.6086, -600.075) -> (-265.6511, -559.1175)
  line L38 (-347.5661, -559.1175) -> (-306.6086, -600.075)
  line L39 (-306.6086, -518.16) -> (-347.5661, -559.1175)
  line L40 (-265.6511, -559.1175) -> (-306.6086, -518.16)
  line L41 (-281.2086, -600.075) -> (-265.6511, -600.075)
  line L42 (-265.6511, -584.5175) -> (-281.2086, -600.075)
  line L43 (-265.6511, -600.075) -> (-265.6511, -584.5175)
  line L44 (-347.5661, -477.2025) -> (-319.3086, -505.46)
  line L45 (-347.5661, -426.4025) -> (-347.5661, -369.8875)
  line L46 (-347.5661, -369.8875) -> (-319.3086, -398.145)
  line L47 (-332.0086, -600.075) -> (-347.5661, -600.075)
  line L48 (-347.5661, -533.7175) -> (-347.5661, -477.2025)
  line L49 (-319.3086, -505.46) -> (-347.5661, -533.7175)
  line L50 (-347.5661, -211.7725) -> (-347.5661, -155.2575)
  line L51 (-347.5661, -88.9) -> (-347.5661, -104.4575)
  line L52 (-319.3086, -183.515) -> (-347.5661, -211.7725)
  line L53 (-347.5661, -584.5175) -> (-332.0086, -600.075)
  line L54 (-347.5661, -262.5725) -> (-319.3086, -290.83)
  line L55 (-347.5661, -155.2575) -> (-319.3086, -183.515)
  line L56 (-347.5661, -319.0875) -> (-347.5661, -262.5725)
  line L57 (-319.3086, -398.145) -> (-347.5661, -426.4025)
  line L58 (-347.5661, -600.075) -> (-347.5661, -584.5175)
  line L59 (-319.3086, -290.83) -> (-347.5661, -319.0875)
  line L60 (-332.0086, -88.9) -> (-347.5661, -88.9)
  line L61 (-347.5661, -104.4575) -> (-332.0086, -88.9)
  dimension "d641" = 45
  dimension "d642" = 12.7
  dimension "d643" = 12.7
  dimension "d645" = 17.9605
  dimension "d646" = 17.9605
  dimension "d710" = 107.315
  dimension "d711" = 0
  dimension "d714" = 107.315
  dimension "d715" = 0
  constraint perpendicular L5 L6
  constraint perpendicular L4 L7
  constraint perpendicular L4 L5
  constraint equal L4 L7
  constraint perpendicular L0 L8
  constraint perpendicular L8 L9
  constraint parallel L7 L10
  constraint coincident L6.end L9
  constraint coincident L4.start L8
  constraint midpoint L1 L11.start
  constraint midpoint L3 L11.end
  constraint coincident L4.start L11
  constraint perpendicular L12 L13
  constraint parallel L11 L14
  constraint parallel L6 L12
  constraint collinear L9 L14
  constraint collinear L5 L13
  constraint midpoint L2 L15.start
  constraint midpoint L0 L15.end
  constraint symmetric L8.start L15 L41.start
  constraint symmetric L8.end L15 L41.end
  constraint symmetric L9.end L15 L42.start
  constraint symmetric L8.start L11 L60.start
  constraint symmetric L8.end L11 L51.start
  constraint symmetric L9.end L11 L51.end
  constraint symmetric L11 L12.start L50.end
  constraint symmetric L11 L12.end L52.start
  constraint symmetric L11 L13.end L50.start
  constraint symmetric L11 L28.start L56.start
  constraint symmetric L11 L28.end L54.start
  constraint symmetric L11 L29.end L54.end
  constraint symmetric L11 L31.start L45.start
  constraint symmetric L11 L31.end L45.end
  constraint symmetric L11 L32.end L46.end
  constraint symmetric L11 L34.start L48.start
  constraint symmetric L11 L34.end L44.start
  constraint symmetric L11 L35.end L44.end
  constraint symmetric L11 L41.start L47.start
  constraint symmetric L11 L41.end L47.end
  constraint symmetric L11 L42.start L53.start
  measures "d641" angle of L2 L4
  measures "d642" distance of L1 L4.start
  measures "d643" distance of L0 L6.end
  measures "d645" distance of L7 L10
  measures "d646" distance of L6 L12
sketch "Sketch4 (3)" plane through (0, 0, 0) normal (-1, 0, 0) x (0, -1, 0) in component "Stretcher"
  line L0 (0, 0) -> (0, 114.3)
  line L1 (0, 114.3) -> (-685.8, 114.3)
  line L2 (-685.8, 114.3) -> (-685.8, 0)
  line L3 (-685.8, 0) -> (0, 0)
  line L4 (-685.8, 57.15) -> (0, 57.15) construction
  line L5 (-342.9, 114.3) -> (-342.9, 0) construction
  line L6 (-673.1, 57.15) -> (-628.65, 101.6)
  line L7 (-628.65, 101.6) -> (-584.2, 57.15)
  line L8 (-584.2, 57.15) -> (-628.65, 12.7)
  line L9 (-628.65, 12.7) -> (-673.1, 57.15)
  line L10 (-673.1, 82.55) -> (-673.1, 101.6)
  line L11 (-673.1, 101.6) -> (-654.05, 101.6)
  line L12 (-654.05, 101.6) -> (-673.1, 82.55)
  line L13 (-603.25, 101.6) -> (-539.75, 101.6)
  line L14 (-539.75, 101.6) -> (-571.5, 69.85)
  line L15 (-571.5, 69.85) -> (-603.25, 101.6)
  line L16 (-514.35, 101.6) -> (-469.9, 57.15)
  line L17 (-469.9, 57.15) -> (-514.35, 12.7)
  line L18 (-514.35, 12.7) -> (-558.8, 57.15)
  line L19 (-558.8, 57.15) -> (-514.35, 101.6)
  line L20 (-400.05, 101.6) -> (-355.6, 57.15)
  line L21 (-355.6, 57.15) -> (-400.05, 12.7)
  line L22 (-400.05, 12.7) -> (-444.5, 57.15)
  line L23 (-444.5, 57.15) -> (-400.05, 101.6)
  line L24 (-285.75, 101.6) -> (-241.3, 57.15)
  line L25 (-241.3, 57.15) -> (-285.75, 12.7)
  line L26 (-285.75, 12.7) -> (-330.2, 57.15)
  line L27 (-330.2, 57.15) -> (-285.75, 101.6)
  line L28 (-171.45, 101.6) -> (-127, 57.15)
  line L29 (-127, 57.15) -> (-171.45, 12.7)
  line L30 (-171.45, 12.7) -> (-215.9, 57.15)
  line L31 (-215.9, 57.15) -> (-171.45, 101.6)
  line L32 (-57.15, 101.6) -> (-12.7, 57.15)
  line L33 (-12.7, 57.15) -> (-57.15, 12.7)
  line L34 (-57.15, 12.7) -> (-101.6, 57.15)
  line L35 (-101.6, 57.15) -> (-57.15, 101.6)
  line L36 (-654.05, 12.7) -> (-673.1, 31.75)
  line L37 (-673.1, 12.7) -> (-654.05, 12.7)
  line L38 (-673.1, 31.75) -> (-673.1, 12.7)
  line L39 (-12.7, 31.75) -> (-12.7, 12.7)
  line L40 (-31.75, 12.7) -> (-12.7, 31.75)
  line L41 (-12.7, 12.7) -> (-31.75, 12.7)
  line L42 (-12.7, 82.55) -> (-12.7, 101.6)
  line L43 (-12.7, 101.6) -> (-31.75, 101.6)
  line L44 (-31.75, 101.6) -> (-12.7, 82.55)
  line L45 (-488.95, 101.6) -> (-425.45, 101.6)
  line L46 (-425.45, 101.6) -> (-457.2, 69.85)
  line L47 (-457.2, 69.85) -> (-488.95, 101.6)
  line L48 (-374.65, 101.6) -> (-311.15, 101.6)
  line L49 (-311.15, 101.6) -> (-342.9, 69.85)
  line L50 (-342.9, 69.85) -> (-374.65, 101.6)
  line L51 (-260.35, 101.6) -> (-196.85, 101.6)
  line L52 (-196.85, 101.6) -> (-228.6, 69.85)
  line L53 (-228.6, 69.85) -> (-260.35, 101.6)
  line L54 (-146.05, 101.6) -> (-82.55, 101.6)
  line L55 (-82.55, 101.6) -> (-114.3, 69.85)
  line L56 (-114.3, 69.85) -> (-146.05, 101.6)
  line L57 (-82.55, 12.7) -> (-114.3, 44.45)
  line L58 (-425.45, 12.7) -> (-457.2, 44.45)
  line L59 (-146.05, 12.7) -> (-82.55, 12.7)
  line L60 (-260.35, 12.7) -> (-196.85, 12.7)
  line L61 (-228.6, 44.45) -> (-260.35, 12.7)
  line L62 (-114.3, 44.45) -> (-146.05, 12.7)
  line L63 (-196.85, 12.7) -> (-228.6, 44.45)
  line L64 (-571.5, 44.45) -> (-603.25, 12.7)
  line L65 (-374.65, 12.7) -> (-311.15, 12.7)
  line L66 (-603.25, 12.7) -> (-539.75, 12.7)
  line L67 (-539.75, 12.7) -> (-571.5, 44.45)
  line L68 (-342.9, 44.45) -> (-374.65, 12.7)
  line L69 (-457.2, 44.45) -> (-488.95, 12.7)
  line L70 (-488.95, 12.7) -> (-425.45, 12.7)
  line L71 (-311.15, 12.7) -> (-342.9, 44.45)
  point P0 (-342.9, 0)
  dimension "d693" = 45
  dimension "d694" = 12.7
  dimension "d695" = 12.7
  dimension "d696" = 17.9605
  dimension "d697" = 17.9605
  dimension "d700" = 114.3
  dimension "d701" = 0
  dimension "d704" = 114.3
  dimension "d705" = 0
  constraint midpoint L2 L4.start
  constraint midpoint L0 L4.end
  constraint midpoint L1 L5.start
  constraint midpoint L3 P0
  constraint coincident L4 L6.start
  constraint coincident L4 L7.end
  constraint parallel L6 L8
  constraint perpendicular L8 L9
  constraint perpendicular L6 L7
  constraint vertical L10
  constraint perpendicular L10 L11
  constraint parallel L6 L12
  constraint coincident L6.end L11
  constraint coincident L6.start L10
  constraint horizontal L13
  constraint parallel L7 L15
  constraint collinear L8 L14
  constraint coincident L6.end L13
  constraint symmetric L4 L10.start L36.end
  constraint symmetric L4 L10.end L37.start
  constraint symmetric L4 L11.end L36.start
  constraint symmetric L5 L10.start L42.start
  constraint symmetric L5 L10.end L42.end
  constraint symmetric L5 L11.end L43.end
  constraint symmetric L5 L36.start L40.start
  constraint symmetric L5 L36.end L39.start
  constraint symmetric L5 L37.start L39.end
  constraint symmetric L4 L5.start P0
  constraint symmetric L4 L13.start L64.end
  constraint symmetric L4 L13.end L66.end
  constraint symmetric L4 L14.end L64.start
  constraint symmetric L4 L45.start L69.end
  constraint symmetric L4 L45.end L58.start
  constraint symmetric L4 L46.end L58.end
  constraint symmetric L4 L48.start L65.start
  constraint symmetric L4 L48.end L65.end
  constraint symmetric L4 L49.end L68.start
  constraint symmetric L4 L51.start L60.start
  constraint symmetric L4 L51.end L60.end
  constraint symmetric L4 L52.end L61.start
  constraint symmetric L4 L54.start L59.start
  constraint symmetric L4 L54.end L57.start
  constraint symmetric L4 L55.end L57.end
  measures "d693" angle of L4 L6
  measures "d694" distance of L4.start L6.start
  measures "d695" distance of L1 L6.end
  measures "d696" distance of L6 L12
  measures "d697" distance of L7 L15
extrude "Extrude4''" [suppressed] in component "Stretcher"
extrude "Extrude6" [suppressed] in component "Panel"
component "TopBoard" placed x (1, 0, 0) y (0, 1, 0) z (0, 0, 1) at (0, 0, 0)
component "BreadBoard" placed x (1, 0, 0) y (0, 1, 0) z (0, 0, 1) at (-195.58, -152.4, 0)
component "TopBoard" placed x (1, 0, 0) y (0, 1, 0) z (0, 0, 1) at (195.58, 0, 0)
component "TopBoard" placed x (1, 0, 0) y (0, 1, 0) z (0, 0, 1) at (391.16, 0, 0)
component "TopBoard_Edge" placed x (1, 0, 0) y (0, 1, 0) z (0, 0, 1) at (-195.58, 0, 0)
component "TopBoard_Edge" placed x (-1, 0, 0) y (0, -1, 0) z (0, 0, 1) at (782.32, 1219.2, 0)
component "BreadBoard" placed x (-1, 0, 0) y (0, -1, 0) z (0, 0, 1) at (782.32, 1371.6, 0)
component "TrestleTop" placed x (1, 0, 0) y (0, 1, 0) z (0, 0, 1) at (-113.03, 228.6, -76.2)
component "TrestleTop" placed x (1, 0, 0) y (0, 1, 0) z (0, 0, 1) at (-113.03, 952.5, -76.2)
component "TrestlePost" placed x (1, 0, 0) y (0, 1, 0) z (0, 0, 1) at (140.97, 228.6, -612.775)
component "TrestlePost" placed x (1, 0, 0) y (0, 1, 0) z (0, 0, 1) at (407.67, 228.6, -612.775)
component "TrestlePost" placed x (1, 0, 0) y (0, 1, 0) z (0, 0, 1) at (140.97, 952.5, -612.775)
component "TrestlePost" placed x (1, 0, 0) y (0, 1, 0) z (0, 0, 1) at (407.67, 952.5, -612.775)
component "TrestleBase" placed x (1, 0, 0) y (0, -1, 0) z (0, 0, -1) at (-113.03, 990.6, -612.775)
component "TrestleBase" placed x (1, 0, 0) y (0, -1, 0) z (0, 0, -1) at (-113.03, 266.7, -612.775)
component "Stretcher" placed x (1, 0, 0) y (0, 1, 0) z (0, 0, 1) at (150.368, 266.7, -241.3)
component "Stretcher" placed x (1, 0, 0) y (0, 1, 0) z (0, 0, 1) at (417.068, 266.7, -241.3)
component "Panel" placed x (1, 0, 0) y (0, 1, 0) z (0, 0, 1) at (-13.2386, 961.898, 0)
component "FloorStretcher" placed x (1, 0, 0) y (0, 1, 0) z (0, 0, 1) at (274.32, -25.4, -688.975)
component "Panel" placed x (1, 0, 0) y (0, 1, 0) z (0, 0, 1) at (-13.2386, 237.998, 0)
equation "length = 60 in"
equation "width = 38.5 in"
equation "height = 28 in"
equation "base_width = 32 in"
equation "base_height = 3 in"
equation "base_thickness = 1.5 in"
equation "top_thickness = 0.875 in"
equation "taper_angle = 9 deg"
equation "taper_distance = ( width - base_width ) / 2"
equation "dovetail_angle = 18 deg"
equation "shoulder_width = 0.25 in"
equation "topBoard_count = 5"
equation "breadboard_width = 6 in"
equation "d18 = length - 2 * breadboard_width"
equation "d19 = top_thickness"
equation "d20 = breadboard_tongueLength"
equation "d21 = top_tenonThickness"
equation "tenon_thickness = 0.5 in"
equation "breadboard_tongueLength = 1 in"
equation "d24 = topBoard_width"
equation "breadboard_tenonLength = breadboard_width - 1 in"
equation "breadboard_tenonWidth = width / topBoard_count / 2"
equation "d28 = breadboard_tenonWidth"
equation "d29 = breadboard_tenonLength - breadboard_tongueLength"
equation "d32 = topBoard_count - 2"
equation "d34 = topBoard_width"
equation "endOverhang = 15 in"
equation "d61 = base_thickness"
equation "d62 = 90 deg + dovetail_angle"
equation "d63 = d62"
equation "d64 = slidingDovetail_depth"
equation "d65 = endOverhang - breadboard_width"
equation "slidingDovetail_depth = ( top_thickness - top_tenonThickness ) / 2"
equation "d18_1 = length - 2 * breadboard_width"
equation "d19_1 = top_thickness"
equation "d20_1 = breadboard_tongueLength"
equation "d21_1 = top_tenonThickness"
equation "d24_1 = topBoard_width"
equation "d28_1 = breadboard_tenonWidth"
equation "d29_1 = breadboard_tenonLength - breadboard_tongueLength"
equation "d61_1 = base_thickness"
equation "d62_1 = 90 deg + dovetail_angle"
equation "d63_1 = d62_1"
equation "d64_1 = slidingDovetail_depth"
equation "d65_1 = endOverhang - breadboard_width"
equation "d73 = slidingDovetail_depth / tan(taper_angle)"
equation "d99 = top_thickness"
equation "d100 = slidingDovetail_depth"
equation "d103 = breadboard_width"
equation "d104 = top_tenonThickness"
equation "d105 = breadboard_tongueLength"
equation "d106 = width"
equation "d108 = breadboard_tenonWidth"
equation "d109 = ( topBoard_width - breadboard_tenonWidth ) / 2"
equation "topBoard_width = width / topBoard_count"
equation "d111 = topBoard_count"
equation "d113 = topBoard_width"
equation "d115 = -( breadboard_tenonLength - breadboard_tongueLength )"
equation "d118 = slidingDovetail_depth"
equation "d146 = base_height"
equation "d147 = base_thickness"
equation "d148 = slidingDovetail_depth"
equation "d149 = 90 deg - dovetail_angle"
equation "d150 = base_width"
equation "d158 = taper_angle"
equation "d159 = trestle_width"
equation "trestle_width = 12 in"
equation "d162 = shoulder_width"
equation "d163 = base_thickness - 2 * shoulder_width"
equation "d164 = tenon_thickness"
equation "panel_thickness = 0.76 in"
equation "d172 = -tenon_length"
equation "tenon_length = 1.5 in"
equation "d199 = base_thickness"
equation "d200 = post_height"
equation "d202 = tenon_thickness"
equation "d203 = shoulder_width"
equation "d204 = tenon_length"
equation "post_height = height - top_thickness - 2 * base_height - foot_thickness"
equation "foot_thickness = 0 in"
equation "d146_1 = base_height"
equation "d147_1 = base_thickness"
equation "d150_1 = base_width"
equation "d158_1 = taper_angle"
equation "d159_1 = trestle_width"
equation "d162_1 = shoulder_width"
equation "d163_1 = base_thickness - 2 * shoulder_width"
equation "d164_1 = tenon_thickness"
equation "d172_1 = -tenon_length"
equation "stretcher_height = post_height - stretcher_width - 2 in"
equation "d337 = tenon_thickness"
equation "d338 = stretcher_width - 2 * shoulder_width"
equation "d339 = stretcher_height + shoulder_width"
equation "d366 = panel_thickness"
equation "d367 = stretcher_width"
equation "d368 = length - 2 * endOverhang - 2 * base_thickness"
equation "d370 = shoulder_width"
equation "d372 = tenon_thickness"
equation "d373 = base_thickness"
equation "d400 = base_thickness"
equation "d401 = wedge_angle"
equation "wedge_angle = 4.5 deg"
equation "d530 = panel_width"
equation "d531 = panel_thickness"
equation "stretcher_width = stretcher_length / 6"
equation "panel_width = post_height / 5"
equation "d559 = panel_width - shoulder_width"
equation "d560 = tenon_thickness"
equation "d561 = tenon_thickness"
equation "d562 = shoulder_width / 2"
equation "d564 = shoulder_width"
equation "d592 = tenon_thickness"
equation "d593 = panel_width - shoulder_width"
equation "top_tenonThickness = 0.25 in"
equation "d595 = taper_angle"
equation "d596 = 90 deg + taper_angle"
equation "d597 = 90 deg + taper_angle"
equation "d599 = -shoulder_width"
equation "d601 = -shoulder_width"
equation "d620 = base_height / 2"
equation "d621 = length - 2 * endOverhang + ( base_width - trestle_width )"